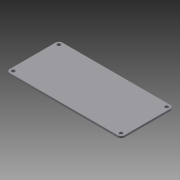
# Autodesk Inventor part: PCB1
Saved by Autodesk Inventor 2015 (Build 190159000, 159)
## iProperties
Created: 2018-03-01
Part Number: PCB1
Material: Generic
Document SubType Name: Modeling
Designer: Silas
Density: 1 g/cm^3
Appearance: Default
Author: Silas
Autodesk Inventor part; units mm, degrees
ref_plane "YZ Plane" through (0, 0, 0) normal (1, 0, 0) x (0, 1, 0)
ref_plane "XZ Plane" through (0, 0, 0) normal (0, 1, 0) x (-1, 0, 0)
ref_plane "XY Plane" through (0, 0, 0) normal (0, 0, 1) x (1, 0, 0)
sketch "Sketch1" plane through (0, 0, 0) normal (0, 0, 1) x (1, 0, 0)
  line L0 (0, 0) -> (99, 0)
  line L1 (99, 0) -> (99, 45.4)
  line L2 (99, 45.4) -> (0, 45.4)
  line L3 (0, 45.4) -> (0, 0)
  circle A0 centre (3, 42.4) radius 1.5
  circle A1 centre (3, 3) radius 1.5
  circle A2 centre (96, 3) radius 1.5
  circle A3 centre (96, 42.4) radius 1.5
  dimension "d0" = 45.4
  dimension "d1" = 99
  dimension "d2" = 3
  dimension "d3" = 3
  dimension "d4" = 3
  dimension "d5" = 3
  dimension "d6" = 3
  dimension "d7" = 3
  dimension "d8" = 3
  dimension "d9" = 3
  dimension "d10" = 3
  dimension "d11" = 3
  dimension "d12" = 3
  dimension "d13" = 3
  constraints: 8 end point, 4 centre point, 2 parallel, 1 horizontal, 1 perpendicular
  measures "d0" distance of L1.end L0.end
  measures "d1" distance of L1.end L2.end
  measures "d2" diameter of A0
  measures "d3" diameter of A1
  measures "d4" diameter of A2
  measures "d5" diameter of A3
  measures "d6" distance from line of L3 A0.centre
  measures "d7" distance from line of L2 A0.centre
  measures "d8" distance from line of L3 A1.centre
  measures "d9" distance from line of L0 A1.centre
  measures "d10" distance from line of L0 A2.centre
  measures "d11" distance from line of L1 A2.centre
  measures "d12" distance from line of L2 A3.centre
  measures "d13" distance from line of L1 A3.centre
extrude "Extrusion1" add sketch "Sketch1" along normal blind 1.6
fillet "Fillet1" radius 3 4 edges at (0, 0, 0.8) (99, 0, 0.8) (99, 45.4, 0.8) (0, 45.4, 0.8)
equation "\"d7\" = d6"
equation "\"d8\" = d9"
equation "\"d9\" = d7"
equation "\"d10\" = d11"
equation "\"d11\" = d8"
equation "\"d12\" = d10"
equation "\"d13\" = d12"
body "Solid1"
